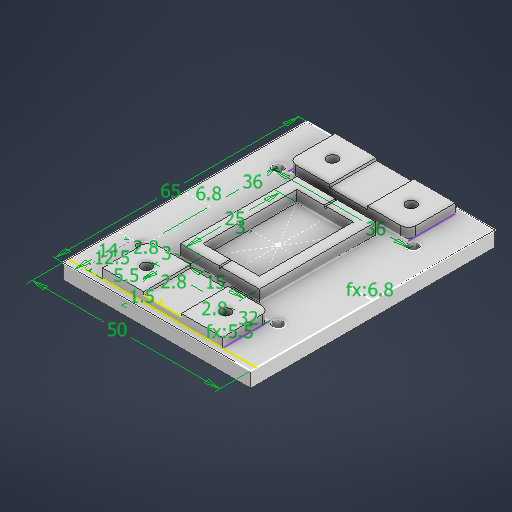
# Autodesk Inventor part: Molde 1FBR 0.5mm
Saved by Autodesk Inventor 2026.1 (Build 301233000, 233)
## iProperties
Created: 2025-07-30
Part Number: Molde 1FBR 0.5mm
Material: Genérico
Document SubType Name: Modeling
Designer: Laboratorio_sensores
Density: 1 g/cm^3
Appearance: Valor por defecto
Author: Laboratorio_sensores
Autodesk Inventor part; units mm, degrees
ref_plane "YZ Plane" through (0, 0, 0) normal (1, 0, 0) x (0, 1, 0)
ref_plane "XZ Plane" through (0, 0, 0) normal (0, 1, 0) x (-1, 0, 0)
ref_plane "XY Plane" through (0, 0, 0) normal (0, 0, 1) x (1, 0, 0)
sketch "Boceto1" plane through (0, 0, 0) normal (0, 1, 0) x (-1, 0, 0)
  line L0 (0, 0) -> (50, 0)
  line L1 (50, 0) -> (50, -65)
  line L2 (50, -65) -> (0, -65)
  line L3 (0, -65) -> (0, 0)
  line L4 (17.7, -45) -> (32.7, -45)
  line L5 (32.7, -45) -> (32.7, -20)
  line L6 (32.7, -20) -> (17.7, -20)
  line L7 (17.7, -20) -> (17.7, -45)
  line L8 (17.7, -45) -> (32.7, -20) construction
  line L9 (32.7, -45) -> (17.7, -20) construction
  line L10 (35.7, -17) -> (35.7, -48)
  line L11 (35.7, -48) -> (14.7, -48)
  line L12 (14.7, -48) -> (14.7, -17)
  line L13 (14.7, -17) -> (35.7, -17)
  line L14 (41, -1.5) -> (9, -1.5)
  line L15 (9, -1.5) -> (9, -14)
  line L16 (9, -14) -> (41, -14)
  line L17 (41, -14) -> (41, -1.5)
  line L18 (32.7, -32.5) -> (17.7, -32.5) construction
  line L19 (41, -7.75) -> (35.5, -7.75) construction
  line L20 (35.5, -7.75) -> (14.5, -7.75) construction
  line L21 (14.5, -7.75) -> (9, -7.75) construction
  circle A0 centre (35.5, -7.75) radius 1.4
  circle A1 centre (14.5, -7.75) radius 1.4
  line L22 (41, -63.5) -> (9, -63.5)
  line L23 (9, -63.5) -> (9, -51)
  line L24 (9, -51) -> (41, -51)
  line L25 (41, -51) -> (41, -63.5)
  circle A2 centre (35.5, -57.25) radius 1.4
  circle A3 centre (14.5, -57.25) radius 1.4
  line L26 (50, -32.5) -> (43.2, -32.5) construction
  line L27 (0, -32.5) -> (6.8, -32.5)
  line L28 (45.9347, 0) -> (45.9347, -14) construction
  line L29 (43.2, -32.5) -> (43.2, -14.5) construction
  line L30 (43.2, -14.5) -> (50, -14.5) construction
  circle A4 centre (43.2, -14.5) radius 1.4
  line L31 (25.2, -20) -> (25.2, -45) construction
  circle A5 centre (7.2, -14.5) radius 1.4
  circle A6 centre (35.5, -57.25) radius 1.4
  circle A7 centre (43.2, -50.5) radius 1.4
  circle A8 centre (7.2, -50.5) radius 1.4
  line L32 (35.5, -7.75) -> (14.5, -7.75)
  point P0 (25.2, -32.5)
  point P1 (25, -14)
  point P2 (25.2, -17)
  dimension "d0" = 65
  dimension "d1" = 50
  dimension "d2" = 25
  dimension "d3" = 15
  dimension "d4" = 3
  dimension "d5" = 12.5
  dimension "d6" = 32
  dimension "d7" = 3
  dimension "d8" = 5.5
  dimension "d9" = 5.5
  dimension "d10" = 2.8
  dimension "d11" = 2.8
  dimension "d12" = 6.8
  dimension "d13" = 6.8
  dimension "d14" = 14
  dimension "d15" = 2.8
  dimension "d30" = 36
  dimension "d31" = 36
  dimension "d32" = 1.5
  constraints: 66 end point, 12 midpoint, 10 symmetric about line, 9 centre point, 8 parallel, 6 horizontal, 5 perpendicular, 3 coincident, 3 point on line, 2 vertical, 1 collinear, 9 other
  measures "d0" distance of L0.end L1.end
  measures "d1" distance of L0.start L0.end
  measures "d2" distance of L4.end L5.end
  measures "d3" distance of L5.end L6.end
  measures "d4" distance between parallel lines of L5 L10
  measures "d5" distance of L16.end L14.start
  measures "d6" distance of L15.end L16.end
  measures "d7" distance between parallel lines of L16 L13
  measures "d8" distance of L19.start L19.end
  measures "d9" distance of L20.end L21.end
  measures "d10" diameter of A0
  measures "d11" diameter of A1
  measures "d12" distance of L26.start L26.end
  measures "d13" distance of L27.start L27.end
  measures "d14" distance of L28.start L28.end
  measures "d15" diameter of A4
  measures "d30" distance of A8.centre A7.centre
  measures "d31" distance of A7.centre L29.end
  measures "d32" distance between parallel lines of L0 L14
extrude "Extrusión1" add sketch "Boceto1" along normal blind 3 contours L10 L11 L12 L13
extrude "Extrusión2" add sketch "Boceto1" against normal blind 4 contours L0 L1 L2 L3 | L17 L16 L15 L14 | L22 L23 L24 L25
extrude "Extrusión3" add sketch "Boceto1" along normal blind 2.5 contours L17 L16 L15 L14 | L22 L23 L24 L25
sketch "Boceto2" plane through (0, 2.5, 0) normal (0, 1, 0) x (1, 0, 0)
  line L0 (-41, 1.5) -> (-9, 1.5) projected
  line L1 (-25, 1.5) -> (-25, 14)
  line L2 (-9, 14) -> (-41, 14) projected
  line L3 (-20, 1.5) -> (-30, 1.5)
  line L4 (-30, 1.5) -> (-30, 14)
  line L5 (-30, 14) -> (-20, 14)
  line L6 (-20, 14) -> (-20, 1.5)
  line L7 (-20, 1.5) -> (-30, 14) construction
  line L8 (-30, 1.5) -> (-20, 14) construction
  line L9 (-32.7, 32.5) -> (-17.7, 32.5) construction
  line L10 (-41, 63.5) -> (-9, 63.5)
  line L11 (-9, 51) -> (-41, 51)
  line L12 (-30, 63.5) -> (-30, 51)
  line L13 (-20, 51) -> (-20, 63.5)
  point P0 (0, 0)
  point P1 (-25, 7.75)
  dimension "d22" = 10
  constraints: 22 end point, 8 symmetric about line, 5 midpoint, 2 parallel, 2 point on line, 1 horizontal, 1 perpendicular
  measures "d22" distance between parallel lines of L4 L6
extrude "Extrusión4" cut sketch "Boceto2" against normal blind 0.75
extrude "Extrusión5" add sketch "Boceto1" against normal blind 4 contours L7 L6 L5 L4 | L10 L11 L12 L13
sketch "Boceto3" plane through (0, 3, 0) normal (0, 1, 0) x (1, 0, 0)
  line L0 (-25.2, 20) -> (-25.2, 45) construction
  line L1 (-35.7, 17) -> (-14.7, 17) projected
  line L2 (-25.2, 17) -> (-25.2, 48)
  line L3 (-14.7, 48) -> (-35.7, 48) projected
  line L4 (-24.95, 17) -> (-25.45, 17)
  line L5 (-25.45, 17) -> (-25.45, 48)
  line L6 (-25.45, 48) -> (-24.95, 48)
  line L7 (-24.95, 48) -> (-24.95, 17)
  line L8 (-24.95, 17) -> (-25.45, 48) construction
  line L9 (-25.45, 17) -> (-24.95, 48) construction
  point P0 (0, 0)
  point P1 (-25.2, 32.5)
  point P2 (-24.95, 17)
  point P3 (-24.95, 48)
  point P4 (-25.45, 17)
  dimension "d27" = 0.5
  constraints: 14 end point, 5 midpoint, 2 parallel, 1 horizontal, 1 perpendicular, 1 point on line
  measures "d27" distance between parallel lines of L5 L7
extrude "Extrusión6" cut sketch "Boceto3" against normal blind 0.5
sketch "Boceto4" plane through (-41, 0, -1.5) normal (0, 0, 1) x (1, 0, 0)
  line L0 (16.05, 2.5) -> (15.55, 2.5) projected
  line L1 (21, 1.75) -> (11, 1.75) projected
  line L2 (-9, 0) -> (41, 0) projected
  line L3 (15.55, 2.5) -> (15.55, 3) projected
fillet "Empalme1" radius 2 4 edges at (-41, 1.25, -51) (-9, 1.25, -51) (-9, 1.25, -14) (-41, 1.25, -14)
equation "\"d9\" = d8"
equation "\"d13\" = d12"
